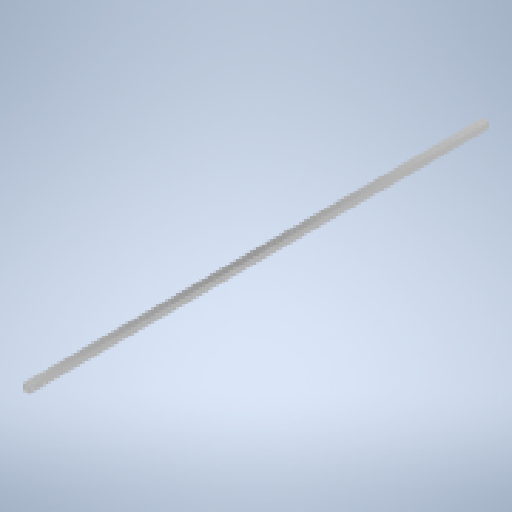
# Autodesk Inventor part: Short tube
Saved by Autodesk Inventor 2024 (Build 280153000, 153)
## iProperties
Created: 2023-04-16
Part Number: Short tube
Material: Aluminum 6061
Document SubType Name: Modeling
Designer: legom
Density: 2.7 g/cm^3
Appearance: Aluminum - Flat
Author: legom
Autodesk Inventor part; units mm, degrees
ref_plane "YZ Plane" through (0, 0, 0) normal (1, 0, 0) x (0, 1, 0)
ref_plane "XZ Plane" through (0, 0, 0) normal (0, 1, 0) x (-1, 0, 0)
ref_plane "XY Plane" through (0, 0, 0) normal (0, 0, 1) x (1, 0, 0)
sketch "Sketch1" plane through (0, 0, 0) normal (0, 0, 1) x (1, 0, 0)
  line L0 (0, 0) -> (25.4, 0)
  line L1 (25.4, 0) -> (25.4, 25.4)
  line L2 (25.4, 25.4) -> (0, 25.4)
  line L3 (0, 25.4) -> (0, 0)
  line L4 (2.286, 23.114) -> (23.114, 23.114)
  line L5 (23.114, 23.114) -> (23.114, 2.286)
  line L6 (23.114, 2.286) -> (2.286, 2.286)
  line L7 (2.286, 2.286) -> (2.286, 23.114)
  dimension "d0" = 25.4
  dimension "d1" = 25.4
  dimension "d2" = 2.286
  constraints: 16 end point, 4 parallel, 2 perpendicular, 1 horizontal, 3 other
  measures "d0" distance of L2.end L1.end
  measures "d1" distance of L1.end L0.end
  measures "d2" distance between parallel lines of L2 L4
extrude "Extrusion1" add sketch "Sketch1" along normal blind 1828.8
sketch "Sketch2" plane through (25.4, 0, 0) normal (0, -1, 0) x (1, 0, 0)
  circle A0 centre (-12.7, 12.7) radius 2.5527
  line L0 (-25.4, 0) -> (-25.4, 1828.8) projected
  line L1 (-25.4, 0) -> (0, 0) projected
  circle A1 centre (-12.7, 38.1) radius 2.5527
  circle A2 centre (-12.7, 63.5) radius 2.5527
  circle A3 centre (-12.7, 88.9) radius 2.5527
  circle A4 centre (-12.7, 114.3) radius 2.5527
  circle A5 centre (-12.7, 139.7) radius 2.5527
  circle A6 centre (-12.7, 165.1) radius 2.5527
  circle A7 centre (-12.7, 190.5) radius 2.5527
  circle A8 centre (-12.7, 215.9) radius 2.5527
  circle A9 centre (-12.7, 241.3) radius 2.5527
  circle A10 centre (-12.7, 266.7) radius 2.5527
  circle A11 centre (-12.7, 292.1) radius 2.5527
  circle A12 centre (-12.7, 317.5) radius 2.5527
  circle A13 centre (-12.7, 342.9) radius 2.5527
  circle A14 centre (-12.7, 368.3) radius 2.5527
  circle A15 centre (-12.7, 393.7) radius 2.5527
  circle A16 centre (-12.7, 419.1) radius 2.5527
  circle A17 centre (-12.7, 444.5) radius 2.5527
  circle A18 centre (-12.7, 469.9) radius 2.5527
  circle A19 centre (-12.7, 495.3) radius 2.5527
  circle A20 centre (-12.7, 520.7) radius 2.5527
  circle A21 centre (-12.7, 546.1) radius 2.5527
  circle A22 centre (-12.7, 571.5) radius 2.5527
  circle A23 centre (-12.7, 596.9) radius 2.5527
  circle A24 centre (-12.7, 622.3) radius 2.5527
  circle A25 centre (-12.7, 647.7) radius 2.5527
  circle A26 centre (-12.7, 673.1) radius 2.5527
  circle A27 centre (-12.7, 698.5) radius 2.5527
  circle A28 centre (-12.7, 723.9) radius 2.5527
  circle A29 centre (-12.7, 749.3) radius 2.5527
  circle A30 centre (-12.7, 774.7) radius 2.5527
  circle A31 centre (-12.7, 800.1) radius 2.5527
  circle A32 centre (-12.7, 825.5) radius 2.5527
  circle A33 centre (-12.7, 850.9) radius 2.5527
  circle A34 centre (-12.7, 876.3) radius 2.5527
  circle A35 centre (-12.7, 901.7) radius 2.5527
  circle A36 centre (-12.7, 927.1) radius 2.5527
  circle A37 centre (-12.7, 952.5) radius 2.5527
  circle A38 centre (-12.7, 977.9) radius 2.5527
  circle A39 centre (-12.7, 1003.3) radius 2.5527
  circle A40 centre (-12.7, 1028.7) radius 2.5527
  circle A41 centre (-12.7, 1054.1) radius 2.5527
  circle A42 centre (-12.7, 1079.5) radius 2.5527
  circle A43 centre (-12.7, 1104.9) radius 2.5527
  circle A44 centre (-12.7, 1130.3) radius 2.5527
  circle A45 centre (-12.7, 1155.7) radius 2.5527
  circle A46 centre (-12.7, 1181.1) radius 2.5527
  circle A47 centre (-12.7, 1206.5) radius 2.5527
  circle A48 centre (-12.7, 1231.9) radius 2.5527
  circle A49 centre (-12.7, 1257.3) radius 2.5527
  circle A50 centre (-12.7, 1282.7) radius 2.5527
  circle A51 centre (-12.7, 1308.1) radius 2.5527
  circle A52 centre (-12.7, 1333.5) radius 2.5527
  circle A53 centre (-12.7, 1358.9) radius 2.5527
  circle A54 centre (-12.7, 1384.3) radius 2.5527
  circle A55 centre (-12.7, 1409.7) radius 2.5527
  circle A56 centre (-12.7, 1435.1) radius 2.5527
  circle A57 centre (-12.7, 1460.5) radius 2.5527
  circle A58 centre (-12.7, 1485.9) radius 2.5527
  circle A59 centre (-12.7, 1511.3) radius 2.5527
  circle A60 centre (-12.7, 1536.7) radius 2.5527
  circle A61 centre (-12.7, 1562.1) radius 2.5527
  circle A62 centre (-12.7, 1587.5) radius 2.5527
  circle A63 centre (-12.7, 1612.9) radius 2.5527
  circle A64 centre (-12.7, 1638.3) radius 2.5527
  circle A65 centre (-12.7, 1663.7) radius 2.5527
  circle A66 centre (-12.7, 1689.1) radius 2.5527
  circle A67 centre (-12.7, 1714.5) radius 2.5527
  circle A68 centre (-12.7, 1739.9) radius 2.5527
  circle A69 centre (-12.7, 1765.3) radius 2.5527
  circle A70 centre (-12.7, 1790.7) radius 2.5527
  circle A71 centre (-12.7, 1816.1) radius 2.5527
  line L2 (-25.4, 1828.8) -> (0, 1828.8)
  line L3 (0, 1828.8) -> (0, 0)
  line L4 (0, 0) -> (-25.4, 0)
  line L5 (-25.4, 0) -> (-25.4, 1828.8)
  dimension "d5" = 5.1054
  dimension "d6" = 12.7
  dimension "d7" = 12.7
  dimension "d10" = 25.4
  constraints: 72 centre point, 8 end point, 2 parallel, 1 horizontal, 1 perpendicular, 1 vertical, 142 other
  measures "d5" diameter of A0
  measures "d6" distance from line of L0 A0.centre
  measures "d7" distance from line of L1 A0.centre
  measures "d10" distance of A0.centre A1.centre
extrude "Extrusion2" cut sketch "Sketch2" against normal through all contours A71
pattern_linear "Rectangular Pattern2" count 73 spacing 25.4 along (0, 0, -1) of "Extrusion2"
sketch "Sketch3" plane through (0, 0, 0) normal (-1, 0, 0) x (0, 0, 1)
  circle A0 centre (1816.1, 12.7) radius 2.5527
  line L0 (1828.8, 25.4) -> (1828.8, 0) projected
  line L1 (0, 25.4) -> (1828.8, 25.4) projected
  circle A1 centre (1790.7, 12.7) radius 2.5527
  circle A2 centre (1765.3, 12.7) radius 2.5527
  circle A3 centre (1012.698, 12.6927) radius 2.5527 projected
  circle A4 centre (1038.098, 12.7) radius 2.5527 projected
  circle A5 centre (1063.498, 12.7073) radius 2.5527 projected
  point P0 (0, 0)
  point P1 (1828.8, 12.7)
  dimension "d23" = 5.1054
  dimension "d24" = 12.7
  dimension "d25" = 12.7
  dimension "d28" = 25.4
  constraints: 3 centre point, 1 horizontal, 1 midpoint, 4 other
  measures "d23" diameter of A0
  measures "d24" distance of point (1828.8, 12.7) A0.centre
  measures "d25" distance from line of L1 A0.centre
  measures "d28" distance of A0.centre A1.centre
extrude "Extrusion3" cut sketch "Sketch3" against normal through all
body "Solid1"
